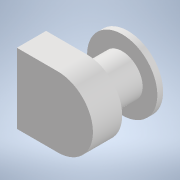
# Autodesk Inventor part: center_holder_top_center
Saved by Autodesk Inventor 2020 (Build 240168000, 168)
## iProperties
Created: 2019-04-30
Part Number: center_holder_top_center
Material: Generic
Document SubType Name: Modeling
Designer: erwin
Density: 1 g/cm^3
Appearance: Default
Author: erwin
Autodesk Inventor part; units mm, degrees
ref_plane "YZ Plane" through (0, 0, 0) normal (1, 0, 0) x (0, 1, 0)
ref_plane "XZ Plane" through (0, 0, 0) normal (0, 1, 0) x (-1, 0, 0)
ref_plane "XY Plane" through (0, 0, 0) normal (0, 0, 1) x (1, 0, 0)
sketch "Sketch1" plane through (0, 0, 0) normal (0, 0, 1) x (1, 0, 0)
  circle A0 centre (-2, 0) radius 4 projected
  arc A1 (-2, 6) -> (-2, -6) centre (-2, 0) ccw projected
  circle A2 centre (-2, 0) radius 6
  line L0 (-2, -6) -> (-9, -6)
  line L1 (-9, -6) -> (-9, 6)
  line L2 (-9, 6) -> (-2, 6)
  line L3 (-2, 6) -> (-2, -6)
  point P0 (0, 0)
  point P1 (-2, -6)
  dimension "d0" = 7
  constraints: 8 end point, 2 parallel, 1 centre point, 1 coincident, 1 concentric, 1 horizontal, 1 perpendicular
  measures "d0" distance of L1.end L2.end
extrude "Extrusion1" add sketch "Sketch1" along normal blind 5
sketch "Sketch2" plane through (0, 0, 0) normal (0, 0, -1) x (-1, 0, 0)
  circle A0 centre (2, 0) radius 4 projected
  circle A1 centre (2, 0) radius 3.5
  point P0 (0, 0)
  dimension "d3" = 7
  constraints: 1 centre point, 1 coincident
  measures "d3" diameter of A1
extrude "Extrusion2" add sketch "Sketch2" along normal blind 6 contours A1
sketch "Sketch4" plane through (-2, 0, -6) normal (0, 0, -1) x (-1, 0, 0)
  circle A0 centre (0, 0) radius 3.5 projected
  point P0 (-2, 0)
  constraints: 1 coincident
hole "Hole1" at (-2, 0, -6) direction (0, 0, 1) diameter 3 end through all
sketch "Sketch5" plane through (-9, -6, 0) normal (0, -1, 0) x (1, 0, 0)
  circle A0 centre (-10.545, -1) radius 4
  circle A1 centre (-10.545, -1) radius 6
  line L0 (0, 0) -> (0, 5) projected
  line L1 (0, 5) -> (-10.545, 5)
  line L2 (0, 5) -> (7, 5) projected
  line L3 (0, 0) -> (7, 0) projected
  line L4 (0, 0) -> (-4.6289, 0)
  point P0 (9, 0)
  dimension "d15" = 8
  dimension "d16" = 12
  constraints: 4 end point, 2 centre point, 2 point on circle, 1 coincident, 1 collinear, 1 horizontal, 1 tangent
  measures "d15" diameter of A0
  measures "d16" diameter of A1
extrude "Extrusion4" add sketch "Sketch5" against normal blind 5
fillet "Fillet1" radius 2 1 edges at (-13.6289, -3.5, 0)
equation "\"d17\" = d1"
equation "\"d1\" = 5"
body "Solid1"
